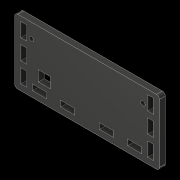
# Autodesk Inventor part: Tester Cheek PE
Saved by Autodesk Inventor 2018 (Build 220112000, 112)
## iProperties
Created: 2017-10-01
Part Number: Tester Cheek PE
Material: UHMW, Black
Document SubType Name: Modeling
Designer: gaine
Density: 0.94 g/cm^3
Appearance: Smooth - Black
Author: gaine
Autodesk Inventor part; units mm, degrees
ref_plane "YZ Plane" through (0, 0, 0) normal (1, 0, 0) x (0, 1, 0)
ref_plane "XZ Plane" through (0, 0, 0) normal (0, 1, 0) x (-1, 0, 0)
ref_plane "XY Plane" through (0, 0, 0) normal (0, 0, 1) x (1, 0, 0)
sketch "Sketch1" plane through (0, 0, 0) normal (0, 0, 1) x (1, 0, 0)
  circle A0 centre (-18.1795, -61.2779) radius 2.413
  circle A1 centre (102.2419, -61.2779) radius 2.413
  line L0 (-23.2595, -45.4029) -> (-23.2595, -64.9896) construction
  line L1 (107.3219, -48.5779) -> (107.3219, -70.0812) construction
  line L2 (116.8469, -45.4029) -> (-32.7845, -45.4029)
  line L3 (120.0219, -48.5779) -> (120.0219, -112.0779)
  line L4 (116.8469, -115.2529) -> (-32.7845, -115.2529)
  line L5 (-35.9595, -112.0779) -> (-35.9595, -48.5779)
  arc A2 (-32.7845, -45.4029) -> (-35.9595, -48.5779) centre (-32.7845, -48.5779) ccw
  arc A3 (-35.9595, -112.0779) -> (-32.7845, -115.2529) centre (-32.7845, -112.0779) ccw
  arc A4 (116.8469, -115.2529) -> (120.0219, -112.0779) centre (116.8469, -112.0779) ccw
  arc A5 (120.0219, -48.5779) -> (116.8469, -45.4029) centre (116.8469, -48.5779) ccw
  line L6 (-29.6095, -50.4829) -> (-23.2595, -50.4829)
  line L7 (-23.2595, -50.4829) -> (-23.2595, -65.7229)
  line L8 (-23.2595, -65.7229) -> (-29.6095, -65.7229)
  line L9 (-29.6095, -65.7229) -> (-29.6095, -50.4829)
  line L10 (-29.6095, -72.0729) -> (-23.2595, -72.0729)
  line L11 (-23.2595, -72.0729) -> (-23.2595, -87.3129)
  line L12 (-23.2595, -87.3129) -> (-29.6095, -87.3129)
  line L13 (-29.6095, -87.3129) -> (-29.6095, -72.0729)
  line L14 (-29.6095, -93.6629) -> (-23.2595, -93.6629)
  line L15 (-23.2595, -93.6629) -> (-23.2595, -108.9029)
  line L16 (-23.2595, -108.9029) -> (-29.6095, -108.9029)
  line L17 (-29.6095, -108.9029) -> (-29.6095, -93.6629)
  line L18 (42.0312, -45.4029) -> (42.0312, -115.2529) construction
  line L19 (113.6719, -50.4829) -> (107.3219, -50.4829)
  line L20 (107.3219, -50.4829) -> (107.3219, -65.7229)
  line L21 (107.3219, -65.7229) -> (113.6719, -65.7229)
  line L22 (113.6719, -65.7229) -> (113.6719, -50.4829)
  line L23 (113.6719, -72.0729) -> (107.3219, -72.0729)
  line L24 (107.3219, -72.0729) -> (107.3219, -87.3129)
  line L25 (107.3219, -87.3129) -> (113.6719, -87.3129)
  line L26 (113.6719, -87.3129) -> (113.6719, -72.0729)
  line L27 (113.6719, -93.6629) -> (107.3219, -93.6629)
  line L28 (107.3219, -93.6629) -> (107.3219, -108.9029)
  line L29 (107.3219, -108.9029) -> (113.6719, -108.9029)
  line L30 (113.6719, -108.9029) -> (113.6719, -93.6629)
  line L31 (-16.9095, -102.5529) -> (-1.6695, -102.5529)
  line L32 (-1.6695, -102.5529) -> (-1.6695, -108.9029)
  line L33 (-1.6695, -108.9029) -> (-16.9095, -108.9029)
  line L34 (-16.9095, -108.9029) -> (-16.9095, -102.5529)
  line L35 (13.5705, -102.5529) -> (28.8105, -102.5529)
  line L36 (28.8105, -102.5529) -> (28.8105, -108.9029)
  line L37 (28.8105, -108.9029) -> (13.5705, -108.9029)
  line L38 (13.5705, -108.9029) -> (13.5705, -102.5529)
  line L39 (100.9719, -102.5529) -> (85.7319, -102.5529)
  line L40 (85.7319, -102.5529) -> (85.7319, -108.9029)
  line L41 (85.7319, -108.9029) -> (100.9719, -108.9029)
  line L42 (100.9719, -108.9029) -> (100.9719, -102.5529)
  line L43 (70.4919, -102.5529) -> (55.2519, -102.5529)
  line L44 (55.2519, -102.5529) -> (55.2519, -108.9029)
  line L45 (55.2519, -108.9029) -> (70.4919, -108.9029)
  line L46 (70.4919, -108.9029) -> (70.4919, -102.5529)
  line L47 (-10.5595, -86.0529) -> (2.4405, -86.0529)
  line L48 (2.4405, -86.0529) -> (2.4405, -97.5529)
  line L49 (2.4405, -97.5529) -> (-10.5595, -97.5529)
  line L50 (-10.5595, -97.5529) -> (-10.5595, -86.0529)
  point P0 (0, 0)
  point P1 (-35.9595, -45.4029)
  point P2 (-35.9595, -115.2529)
  point P3 (107.3219, -64.9896)
  dimension "d3" = 4.826
  dimension "d4" = 4.826
  dimension "d7" = 120.4214
  dimension "d8" = 5.08
  dimension "d9" = 5.08
  dimension "d18" = 15.875
  dimension "d19" = 15.875
  dimension "d20" = 90
  dimension "d21" = 12.7
  dimension "d22" = 155.9814
  dimension "d23" = 69.85
  dimension "d24" = 3.175
  dimension "d25" = 6.35
  dimension "d26" = 6.35
  dimension "d27" = 15.24
  dimension "d28" = 15.24
  dimension "d29" = 15.24
  dimension "d30" = 6.35
  dimension "d31" = 6.35
  dimension "d32" = 6.35
  dimension "d37" = 15.24
  dimension "d38" = 15.24
  dimension "d40" = 6.35
  dimension "d41" = 15.24
  dimension "d50" = 6.35
  dimension "d53" = 11.5
  dimension "d54" = 13
  dimension "d55" = 5
  dimension "d56" = 12.7
  constraints: 102 end point, 21 symmetric about line, 12 parallel, 10 point on line, 8 point on circle, 8 tangent, 7 horizontal, 7 perpendicular, 6 centre point, 4 collinear, 3 equal radius, 2 midpoint, 1 vertical
  measures "d3" diameter of A0
  measures "d4" diameter of A1
  measures "d7" distance of A0.centre A1.centre
  measures "d8" distance from line of L0 A0.centre
  measures "d9" distance from line of L1 A1.centre
  measures "d18" distance from line of L2 A0.centre
  measures "d19" distance from line of L2 A1.centre
  measures "d20" angle of L3 L2
  measures "d21" distance between parallel lines of L5 L0
  measures "d22" distance between parallel lines of L3 L5
  measures "d23" distance of point (-35.959, -115.253) point (-35.959, -45.403)
  measures "d24" radius of A2
  measures "d25" distance between parallel lines of L9 L7
  measures "d26" distance between parallel lines of L5 L9
  measures "d27" distance between parallel lines of L14 L16
  measures "d28" distance between parallel lines of L10 L12
  measures "d29" distance between parallel lines of L6 L8
  measures "d30" distance between parallel lines of L4 L16
  measures "d31" distance between parallel lines of L12 L14
  measures "d32" distance between parallel lines of L8 L10
  measures "d37" distance between parallel lines of L32 L34
  measures "d38" distance between parallel lines of L36 L38
  measures "d40" distance between parallel lines of L15 L34
  measures "d41" distance between parallel lines of L38 L32
  measures "d50" distance between parallel lines of L33 L31
  measures "d53" distance between parallel lines of L49 L47
  measures "d54" distance between parallel lines of L48 L50
  measures "d55" distance between parallel lines of L31 L49
  measures "d56" distance between parallel lines of L15 L50
extrude "Extrusion6" add sketch "Sketch1" along normal blind 6.35
equation "\"d4\" = d3"
equation "\"d19\" = d18"
equation "\"d22\" = 2 * d21 + d7 + d9 + d8"
equation "\"d28\" = d27"
equation "\"d29\" = d27"
equation "\"d31\" = d30"
equation "\"d32\" = d30"
equation "\"d37\" = d27"
equation "\"d38\" = d27"
equation "\"d40\" = d30"
body "Solid5"
